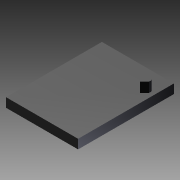
# Autodesk Inventor part: B12APblack
Saved by Autodesk Inventor 2011 SP1 (Build 150282100, 282)
## iProperties
Created: 2013-12-24
Part Number: B12APblack
Catalog Web Link: www.cadenas.de
Description: B Series - Black Body-
Vendor: NKKSWITCHES
Document SubType Name: Modeling
Designer: PARTuser1
Manufacturer: NKKSWITCHES
Density: 1 g/cm^3
Category: PARTsolutions
Company: NKKSWITCHES
Title: B12APblack
Author: Cadenas PARTsolutions
PSOL_IDENT_0: {$CADENAS_DATA\23d-libs\nkkswitches\toggle\b\parts\b_black_body.prj},199 {VTYP=3D},{NB=B12APblack},{
PSOL_IDENT_1: LINA=B12APblack},{NN=B Series - Black Body},{DATE=06.03.2009 07:32:26},{GEOMDATE=02.02.2009 08:55:00
PSOL_IDENT_2: },{VERSION=},{LINEID=10},{LINESUBID=-1},{WBVAR=PLS,CRCTS,TGGLS,TRMNLS}  {NB=B12APblack},{LINA=B12APb
PSOL_IDENT_3: lack},{KT=DUMMY},{PN=B12AP},{SRS=B},{PLS=1},{CRCTS=2},{CRCTSALG= '2','2 - ON/NONE/ON','3','3 - ON/OF
PSOL_IDENT_4: F/ON','5','5 - ON/NONE/(ON)','R','R - (ON)/NONE/ON','8','8 - (ON)/OFF/(ON)','9','9 - ON/OFF/(ON)','S
PSOL_IDENT_5: ','S - (ON)/OFF/ON' },{TGGLS=A},{TGGLSALG=  'A','A - .394\" (10.0 mm) Bat','J','J - .248\" (6.3 mm)
PSOL_IDENT_6: Bat','E','E - .394\" (10.0 mm) Flatted','H','H - .248\" (6.3 mm) Flatted','K','K - Snap Top for Padd
PSOL_IDENT_7: les' },{TRMNLS=P},{TRMNLSALG= 'P','P - Straight','B','B - Straight with Bracket', 'H','H - Right Ang
PSOL_IDENT_8: le with Bracket','V','V - Vertical with Bracket' ,'W','W - Straight Long' }
CNS_NN: B Series - Black Body
CNS_NB: B12APblack
CNS_NBSYN: $PN.black
CNS_LINA: B12APblack
CNS_PN: B12AP
CNS_SRS: B
CNS_PLS: 1 - SPDT
CNS_CRCTS: 2 - ON/NONE/ON
CNS_CRCTSALG: '2','2 - ON/NONE/ON','3','3 - ON/OFF/ON','5','5 - ON/NONE/(ON)','R','R - (ON)/NONE/ON','8','8 - (ON)/OFF/(ON)','9','9 - ON/OFF/(ON)','S','S - (ON)/OFF/ON'
CNS_TGGLS: A - .394" (10.0 mm) Bat
CNS_TGGLSALG: 'A','A - .394" (10.0 mm) Bat','J','J - .248" (6.3 mm) Bat','E','E - .394" (10.0 mm) Flatted','H','H - .248" (6.3 mm) Flatted','K','K - Snap Top for Paddles'
CNS_TRMNLS: P - Straight
CNS_TRMNLSALG: 'P','P - Straight','B','B - Straight with Bracket', 'H','H - Right Angle with Bracket','V','V - Vertical with Bracket' ,'W','W - Straight Long'
SUPPLIER: NKKSWITCHES
ARTICLENO: B12APblack
BOMINFO: B12APblack
CREATOR: CADENAS GmbH
Autodesk Inventor part; units mm, degrees
sketch "Sketch_1" plane through (0, 0, 0) normal (0, 1, 0) x (-1, 0, 0)
  line L0 (2.9972, 3.9878) -> (-2.9972, 3.9878)
  line L1 (-2.9972, 3.9878) -> (-2.9972, -3.9878)
  line L2 (-2.9972, -3.9878) -> (2.9972, -3.9878)
  line L3 (2.9972, -3.9878) -> (2.9972, 3.9878)
  constraints: 8 end point
extrude "Extrusion1" add sketch "Sketch_1" along normal blind 0.762
sketch "Sketch_11" plane through (0, 0.762, 0) normal (0, 1, 0) x (1, 0, 0)
  arc A0 (2.2553, 1.8961) -> (1.8961, 2.2553) centre (0, 0) ccw
  line L0 (2.2553, 1.8961) -> (2.6313, 2.2721)
  arc A1 (2.6313, 2.2721) -> (2.2721, 2.6313) centre (2.3718, 2.3718) ccw
  line L1 (2.2721, 2.6313) -> (1.8961, 2.2553)
  constraints: 4 end point, 4 point on circle, 2 centre point
extrude "Extrusion2" add sketch "Sketch_11" along normal blind 0.8128
ref_plane "cp_body_raiv_XY" through (0, 0, 0) normal (0, 0, 1) x (1, 0, 0)
ref_plane "cp_body_raiv_YZ" through (0, 0, 0) normal (1, 0, 0) x (0, 1, 0)
ref_plane "cp_body_raiv_ZX" through (0, 0, 0) normal (0, 1, 0) x (0, 0, 1)
ref_plane "cp_body_str_XY" through (0, 0, 0) normal (0, 1, 0) x (1, 0, 0)
ref_plane "cp_body_str_YZ" through (0, 0, 0) normal (1, 0, 0) x (0, 0, -1)
ref_plane "cp_body_str_ZX" through (0, 0, 0) normal (0, 0, -1) x (0, 1, 0)
ref_plane "cp_body_togg_rv_XY" through (0, 0, 0.762) normal (0, 0, -1) x (1, 0, 0)
ref_plane "cp_body_togg_rv_YZ" through (0, 0, 0.762) normal (1, 0, 0) x (0, -1, 0)
ref_plane "cp_body_togg_rv_ZX" through (0, 0, 0.762) normal (0, -1, 0) x (0, 0, -1)
ref_plane "cp_body_togstr_XY" through (0, 0.762, 0) normal (0, -1, 0) x (1, 0, 0)
ref_plane "cp_body_togstr_YZ" through (0, 0.762, 0) normal (1, 0, 0) x (0, 0, 1)
ref_plane "cp_body_togstr_ZX" through (0, 0.762, 0) normal (0, 0, 1) x (0, -1, 0)
body "Solid1"
